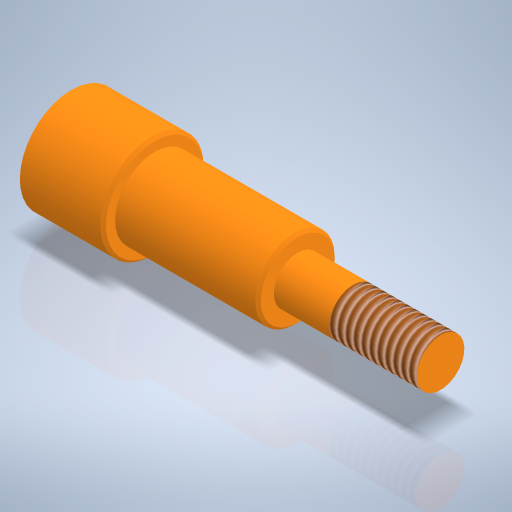
# Autodesk Inventor part: 102
Saved by Autodesk Inventor 2024 (Build 280153000, 153)
## iProperties
Created: 2024-07-12
Part Number: 102
Material: Silber
Document SubType Name: Modeling
Designer: ffogue
Density: 10.49 g/cm^3
Appearance: Orange
Author: ffogue
Autodesk Inventor part; units mm, degrees
ref_plane "YZ Plane" through (0, 0, 0) normal (1, 0, 0) x (0, 1, 0)
ref_plane "XZ Plane" through (0, 0, 0) normal (0, 1, 0) x (-1, 0, 0)
ref_plane "XY Plane" through (0, 0, 0) normal (0, 0, 1) x (1, 0, 0)
sketch "Skizze1" plane through (0, 0, 0) normal (0, 1, 0) x (-1, 0, 0)
  line L0 (0, 0) -> (0, 6.5)
  line L1 (0, 6.5) -> (-10.5, 6.5)
  line L2 (-10.5, 6.5) -> (-10.5, 5)
  line L3 (-10.5, 5) -> (-28.5, 5)
  line L4 (-28.5, 5) -> (-28.5, 3)
  line L5 (-28.5, 3) -> (-46.5, 3)
  line L6 (-46.5, 3) -> (-46.5, 0)
  line L7 (-46.5, 0) -> (0, 0)
  dimension "d0" = 46.5
  dimension "d1" = 13
  dimension "d2" = 10
  dimension "d3" = 6
  dimension "d4" = 10.5
  dimension "d5" = 18
  constraints: 16 end point, 7 perpendicular, 1 vertical
  measures "d0" distance between parallel lines of L6 L0
  measures "d1" diameter of L1 L7
  measures "d2" diameter of L3 L7
  measures "d3" diameter of L5 L7
  measures "d4" distance between parallel lines of L2 L0
  measures "d5" distance between parallel lines of L4 L2
revolve "Umdrehung1" add sketch "Skizze1" angle 360 about axis through (46.5, 0, 0) along (-1, 0, 0)
thread "Gewinde1" size "M6x1" class "6g" standard "ISO Metric profile" length 11
sketch "Skizze2" plane through (0, 0, 0) normal (-1, 0, 0) x (0, 0, 1)
  circle A0 centre (0, 0) radius 6.5 projected
  point P0 (0, 0)
  constraints: 1 coincident
hole "Bohrung1" at (0, 0, 0) direction (1, 0, 0) diameter 4 depth 26
chamfer "Fasen1" distance 0.35 angle 45 2 edges at (28.5, 0, -5) (10.5, 0, -6.5)
